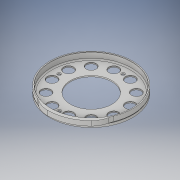
# Autodesk Inventor part: Component 19 (Rear Cam Disc)
Saved by Autodesk Inventor 2018 (Build 220112000, 112)
## iProperties
Created: 2023-03-15
Part Number: Component 19 (Rear Cam Disc)
Material: Generic
Document SubType Name: Modeling
Designer: Habib Mohamed
Density: 1 g/cm^3
Appearance: Default
Author: Habib Mohamed
Autodesk Inventor part; units mm, degrees
ref_plane "YZ Plane" through (0, 0, 0) normal (1, 0, 0) x (0, 1, 0)
ref_plane "XZ Plane" through (0, 0, 0) normal (0, 1, 0) x (-1, 0, 0)
ref_plane "XY Plane" through (0, 0, 0) normal (0, 0, 1) x (1, 0, 0)
sketch "Sketch1" plane through (0, 0, 0) normal (0, 1, 0) x (-1, 0, 0)
  circle A0 centre (0, 0) radius 17.5
  circle A1 centre (0, 0) radius 34
  circle A2 centre (0, 0) radius 35
  circle A3 centre (0, 0) radius 36 construction
  arc A4 (10.3, 33.97) -> (11.84, 33.07) centre (21.1513, 50.7703) ccw
  arc A5 (10.3, 33.97) -> (0, 37) centre (0.0064, 18) ccw
  arc A6 (0, 37) -> (-26.16, 26.16) centre (0.0059, 0) ccw
  arc A7 (-26.16, 26.16) -> (-31.3, 16.74) centre (-12.7302, 12.7197) ccw
  arc A8 (-32.359, 13.3377) -> (-31.3, 16.74) centre (-50.8499, 20.9592) ccw
  arc A9 (11.84, 33.07) -> (13.4398, 32.3167) centre (21.1513, 50.7703) ccw
  point P0 (-32.36, 13.335)
  dimension "d0" = 35
  dimension "d1" = 68
  dimension "d2" = 70
  dimension "d3" = 72
  dimension "d4" = 32.36
  dimension "d5" = 1.06
  dimension "d6" = 5.14
  dimension "d7" = 26.16
  dimension "d8" = 10.3
  dimension "d9" = 1.54
  dimension "d10" = 16.74
  dimension "d11" = 26.16
  dimension "d12" = 37
  dimension "d13" = 33.97
  dimension "d14" = 33.07
  dimension "d15" = 13.335
  dimension "d16" = 20
  dimension "d17" = 19
  dimension "d18" = 37
  dimension "d19" = 19
  dimension "d20" = 20
  dimension "d21" = 20
  constraints: 14 point on circle, 10 centre point, 5 coincident, 2 tangent
  measures "d0" diameter of A0
  measures "d1" diameter of A1
  measures "d2" diameter of A2
  measures "d3" diameter of A3
  measures "d4" horizontal distance of point (-32.36, 13.335) point (0, 0)
  measures "d5" horizontal distance of A7.end point (-32.36, 13.335)
  measures "d6" horizontal distance of point (-26.16, 26.16) A7.end
  measures "d7" horizontal distance of A5.end point (-26.16, 26.16)
  measures "d8" horizontal distance of A5.end A4.start
  measures "d9" horizontal distance of A4.end A4.start
  measures "d10" vertical distance of A7.end point (0, 0)
  measures "d11" horizontal distance of point (0, 0) point (-26.16, 26.16)
  measures "d12" distance of point (0, 0) A5.end
  measures "d13" vertical distance of point (0, 0) A4.start
  measures "d14" vertical distance of point (0, 0) A4.end
  measures "d15" vertical distance of point (0, 0) point (-32.36, 13.335)
  measures "d16" radius of A4
  measures "d17" radius of A5
  measures "d18" radius of A6
  measures "d19" radius of A7
  measures "d20" radius of A8
  measures "d21" radius of A9
extrude "Extrusion1" add sketch "Sketch1" along normal blind 6.5 contours A1 | A2 | A2 A8 A7 A6 A5 A4 A9
extrude "Extrusion2" cut sketch "Sketch1" against normal blind 5.5 from surface at 6.5 contours A1
extrude "Extrusion3" cut sketch "Sketch1" along normal blind 2.5 contours A2 A8 A7 A6 A5 A4 A9
sketch "Sketch2" plane through (0, 0, 0) normal (1, 0, 0) x (0, 1, 0)
  line L0 (0, -35) -> (0, -17.5) projected
  line L1 (0, -17.5) -> (1, -17.5) projected
  line L2 (1, -17.5) -> (1, -34) projected
  line L3 (1, -34) -> (6.5, -34) projected
  line L4 (6.5, -34) -> (6.5, -35) projected
  line L5 (6.5, -35) -> (0, -35) projected
  line L6 (0, 17.5) -> (0, 35) projected
  line L7 (0, 35) -> (2.5, 35) projected
  line L8 (2.5, 35) -> (2.5, 37) projected
  line L9 (2.5, 37) -> (6.5, 37) projected
  line L10 (6.5, 37) -> (6.5, 34) projected
  line L11 (6.5, 34) -> (1, 34) projected
  line L12 (1, 34) -> (1, 17.5) projected
  line L13 (1, 17.5) -> (0, 17.5) projected
  line L14 (0, 35) -> (2.5, 35) projected
  line L15 (2.5, 35) -> (2, 35)
  line L16 (2, 35) -> (2, 34.75)
  line L17 (2, 34.75) -> (2.5, 34.75)
  line L18 (2.5, 34.75) -> (2.5, 35)
  line L19 (0, 0) -> (15.0965, 0) construction
  dimension "d28" = 0.5
  dimension "d29" = 2
  dimension "d30" = 0.25
  constraints: 10 end point, 2 horizontal, 2 parallel, 1 perpendicular, 1 point on line
  measures "d28" distance of L16.end L17.end
  measures "d29" distance between parallel lines of L6 L16
  measures "d30" distance of L15.end L16.end
revolve "Revolution1" cut sketch "Sketch2" angle 360 about axis through (0, 0, 0) along (0, 1, 0) contours L7 L18 L17 L16
sketch "Sketch3" plane through (0, 1, 0) normal (0, 1, 0) x (1, 0, 0)
  circle A0 centre (0, 0) radius 27 construction
  point P0 (-27, 0)
  point P1 (-26.0795, 6.99)
  dimension "d32" = 54
  dimension "d33" = 27
  dimension "d35" = 6.99
  constraints: 1 centre point, 1 coincident, 1 horizontal alignment, 1 point on circle
  measures "d32" diameter of A0
  measures "d33" distance of point (0, 0) A0.start
  measures "d35" vertical distance of A0.end A0.start
hole "Hole1" at (-26.0795, 1, -6.99) direction (0, -1, 0) diameter 8 end through all
hole "Hole2" at (-27, 1, 0) direction (0, -1, 0) diameter 2 end through all
chamfer "Chamfer1" distance 0.5 angle 45 1 edges at (-27, 1, -1)
chamfer "Chamfer2" distance 0.2 angle 45 1 edges at (-26.0795, 1, -10.99)
pattern_circular "Circular Pattern1" count 12 over 360 about axis through (0, 0, 0) along (0, -1, 0) of "Hole1", "Chamfer2"
pattern_circular "Circular Pattern2" count 3 over 180 about axis through (0, 0, 0) along (0, -1, 0) of "Hole2", "Chamfer1" both ways yes
fillet "Fillet1" radius 1 1 edges at (34, 1, 0)
fillet "Fillet2" radius 0.2 1 edges at (34, 6.5, 0)
equation "\"d41\" = d33"
equation "\"d48\" = d33"
body "Solid1"
